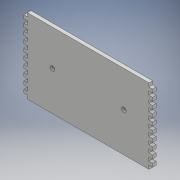
# Autodesk Inventor part: Base
Saved by Autodesk Inventor 2017 (Build 210142000, 142)
## iProperties
Created: 2017-04-26
Part Number: Base
Material: Generic
Document SubType Name: Modeling
Designer: Parshant Bombhi
Density: 1 g/cm^3
Appearance: Default
Author: Parshant Bombhi
Autodesk Inventor part; units mm, degrees
ref_plane "YZ Plane" through (0, 0, 0) normal (1, 0, 0) x (0, 1, 0)
ref_plane "XZ Plane" through (0, 0, 0) normal (0, 1, 0) x (-1, 0, 0)
ref_plane "XY Plane" through (0, 0, 0) normal (0, 0, 1) x (1, 0, 0)
sketch "Sketch5" plane through (0, 0, 0) normal (0, 1, 0) x (-1, 0, 0)
  circle A0 centre (177.8, -63.5) radius 3.9688
  circle A1 centre (50.8, -63.5) radius 3.9687
  line L0 (6.35, 0) -> (6.35, -6.35)
  line L1 (6.35, -6.35) -> (0, -6.35)
  line L2 (0, -6.35) -> (0, -12.7)
  line L3 (0, -12.7) -> (6.35, -12.7)
  line L4 (6.35, -12.7) -> (6.35, -19.05)
  line L5 (6.35, -19.05) -> (0, -19.05)
  line L6 (0, -19.05) -> (0, -25.4)
  line L7 (0, -25.4) -> (6.35, -25.4)
  line L8 (6.35, -25.4) -> (6.35, -31.75)
  line L9 (6.35, -31.75) -> (0, -31.75)
  line L10 (0, -31.75) -> (0, -38.1)
  line L11 (0, -38.1) -> (6.35, -38.1)
  line L12 (6.35, -38.1) -> (6.35, -44.45)
  line L13 (6.35, -44.45) -> (0, -44.45)
  line L14 (0, -44.45) -> (0, -50.8)
  line L15 (0, -50.8) -> (6.35, -50.8)
  line L16 (6.35, -50.8) -> (6.35, -57.15)
  line L17 (6.35, -57.15) -> (0, -57.15)
  line L18 (0, -57.15) -> (0, -63.5)
  line L19 (0, -63.5) -> (6.35, -63.5)
  line L20 (6.35, -63.5) -> (6.35, -69.85)
  line L21 (6.35, -69.85) -> (0, -69.85)
  line L22 (0, -69.85) -> (0, -76.2)
  line L23 (0, -76.2) -> (6.35, -76.2)
  line L24 (6.35, -76.2) -> (6.35, -82.55)
  line L25 (6.35, -82.55) -> (0, -82.55)
  line L26 (0, -82.55) -> (0, -88.9)
  line L27 (0, -88.9) -> (6.35, -88.9)
  line L28 (6.35, -88.9) -> (6.35, -95.25)
  line L29 (6.35, -95.25) -> (0, -95.25)
  line L30 (0, -95.25) -> (0, -101.6)
  line L31 (0, -101.6) -> (6.35, -101.6)
  line L32 (6.35, -101.6) -> (6.35, -107.95)
  line L33 (6.35, -107.95) -> (0, -107.95)
  line L34 (0, -107.95) -> (0, -114.3)
  line L35 (0, -114.3) -> (6.35, -114.3)
  line L36 (6.35, -114.3) -> (6.35, -120.65)
  line L37 (6.35, -120.65) -> (0, -120.65)
  line L38 (0, -120.65) -> (0, -127)
  line L39 (0, -127) -> (6.35, -127)
  line L40 (6.35, -127) -> (6.35, -133.35)
  line L41 (222.25, -133.35) -> (222.25, -127)
  line L42 (222.25, -127) -> (228.6, -127)
  line L43 (228.6, -127) -> (228.6, -120.65)
  line L44 (228.6, -120.65) -> (222.25, -120.65)
  line L45 (222.25, -120.65) -> (222.25, -114.3)
  line L46 (222.25, -114.3) -> (228.6, -114.3)
  line L47 (228.6, -114.3) -> (228.6, -107.95)
  line L48 (228.6, -107.95) -> (222.25, -107.95)
  line L49 (222.25, -107.95) -> (222.25, -101.6)
  line L50 (222.25, -101.6) -> (228.6, -101.6)
  line L51 (228.6, -101.6) -> (228.6, -95.25)
  line L52 (228.6, -95.25) -> (222.25, -95.25)
  line L53 (222.25, -95.25) -> (222.25, -88.9)
  line L54 (222.25, -88.9) -> (228.6, -88.9)
  line L55 (228.6, -88.9) -> (228.6, -82.55)
  line L56 (228.6, -82.55) -> (222.25, -82.55)
  line L57 (222.25, -82.55) -> (222.25, -76.2)
  line L58 (222.25, -76.2) -> (228.6, -76.2)
  line L59 (228.6, -76.2) -> (228.6, -69.85)
  line L60 (228.6, -69.85) -> (222.25, -69.85)
  line L61 (222.25, -69.85) -> (222.25, -63.5)
  line L62 (222.25, -63.5) -> (228.6, -63.5)
  line L63 (228.6, -63.5) -> (228.6, -57.15)
  line L64 (228.6, -57.15) -> (222.25, -57.15)
  line L65 (222.25, -57.15) -> (222.25, -50.8)
  line L66 (222.25, -50.8) -> (228.6, -50.8)
  line L67 (228.6, -50.8) -> (228.6, -44.45)
  line L68 (228.6, -44.45) -> (222.25, -44.45)
  line L69 (222.25, -44.45) -> (222.25, -38.1)
  line L70 (222.25, -38.1) -> (228.6, -38.1)
  line L71 (228.6, -38.1) -> (228.6, -31.75)
  line L72 (228.6, -31.75) -> (222.25, -31.75)
  line L73 (222.25, -31.75) -> (222.25, -25.4)
  line L74 (222.25, -25.4) -> (228.6, -25.4)
  line L75 (228.6, -25.4) -> (228.6, -19.05)
  line L76 (228.6, -19.05) -> (222.25, -19.05)
  line L77 (222.25, -19.05) -> (222.25, -12.7)
  line L78 (222.25, -12.7) -> (228.6, -12.7)
  line L79 (228.6, -12.7) -> (228.6, -6.35)
  line L80 (228.6, -6.35) -> (222.25, -6.35)
  line L81 (222.25, -6.35) -> (222.25, 0)
  line L82 (6.35, 0) -> (222.25, 0)
  line L83 (222.25, -133.35) -> (6.35, -133.35)
  point P0 (0, 0)
  dimension "Shaft_Diameter" = 7.9375
  dimension "d59" = 7.9375
  dimension "d73" = 6.35
  dimension "Teeth_Width" = 6.35
  dimension "d79" = 6.35
  dimension "d80" = 6.35
  dimension "d81" = 6.35
  dimension "d82" = 6.35
  dimension "d92" = 6.35
  dimension "d93" = 6.35
  dimension "d94" = 6.35
  dimension "d95" = 6.35
  dimension "d96" = 6.35
  dimension "d97" = 6.35
  dimension "d100" = 6.35
  dimension "d101" = 6.35
  dimension "d102" = 6.35
  dimension "d103" = 6.35
  dimension "d106" = 6.35
  dimension "d107" = 6.35
  dimension "d108" = 6.35
  dimension "d109" = 6.35
  dimension "d112" = 6.35
  dimension "d113" = 6.35
  dimension "d114" = 6.35
  dimension "d115" = 6.35
  dimension "d118" = 6.35
  dimension "d119" = 6.35
  dimension "d120" = 6.35
  dimension "d121" = 6.35
  dimension "d124" = 6.35
  dimension "d125" = 6.35
  dimension "d126" = 6.35
  dimension "d127" = 6.35
  dimension "d130" = 6.35
  dimension "d131" = 6.35
  dimension "d132" = 6.35
  dimension "d133" = 6.35
  dimension "d136" = 6.35
  dimension "d137" = 6.35
  dimension "d138" = 6.35
  dimension "d139" = 6.35
  dimension "d143" = 6.35
  dimension "d149" = 6.35
  dimension "d150" = 6.35
  dimension "d151" = 6.35
  dimension "d152" = 6.35
  dimension "d153" = 6.35
  dimension "d154" = 6.35
  dimension "d155" = 6.35
  dimension "d156" = 6.35
  dimension "d157" = 6.35
  dimension "d158" = 6.35
  dimension "d159" = 6.35
  dimension "d160" = 6.35
  dimension "d161" = 6.35
  dimension "d162" = 6.35
  dimension "d163" = 6.35
  dimension "d164" = 6.35
  dimension "d165" = 6.35
  dimension "d166" = 6.35
  dimension "d167" = 6.35
  dimension "d168" = 6.35
  dimension "d169" = 6.35
  constraints: 168 end point, 60 perpendicular, 11 horizontal, 11 vertical, 2 centre point
  measures "Shaft_Diameter" diameter of A0
  measures "d59" diameter of A1
  measures "d73" distance of L1.end L2.end
  measures "Teeth_Width" distance of L0.start L0.end
  measures "d79" distance between parallel lines of L0 L2
  measures "d80" distance of L5.end L6.end
  measures "d81" distance of L3.end L4.end
  measures "d82" distance between parallel lines of L4 L6
  measures "d92" distance of L6.end L7.end
  measures "d93" distance between parallel lines of L2 L4
  measures "d94" distance of L9.end L10.end
  measures "d95" distance of L7.end L8.end
  measures "d96" distance between parallel lines of L8 L10
  measures "d97" distance of L10.end L11.end
  measures "d100" distance of L13.end L14.end
  measures "d101" distance of L11.end L12.end
  measures "d102" distance between parallel lines of L12 L14
  measures "d103" distance of L14.end L15.end
  measures "d106" distance of L17.end L18.end
  measures "d107" distance of L15.end L16.end
  measures "d108" distance between parallel lines of L16 L18
  measures "d109" distance of L18.end L19.end
  measures "d112" distance of L21.end L22.end
  measures "d113" distance of L19.end L20.end
  measures "d114" distance between parallel lines of L20 L22
  measures "d115" distance of L22.end L23.end
  measures "d118" distance of L25.end L26.end
  measures "d119" distance of L23.end L24.end
  measures "d120" distance between parallel lines of L24 L26
  measures "d121" distance of L26.end L27.end
  measures "d124" distance of L29.end L30.end
  measures "d125" distance of L27.end L28.end
  measures "d126" distance between parallel lines of L28 L30
  measures "d127" distance of L30.end L31.end
  measures "d130" distance of L33.end L34.end
  measures "d131" distance of L31.end L32.end
  measures "d132" distance between parallel lines of L32 L34
  measures "d133" distance of L34.end L35.end
  measures "d136" distance of L37.end L38.end
  measures "d137" distance of L35.end L36.end
  measures "d138" distance between parallel lines of L36 L38
  measures "d139" distance of L38.end L39.end
  measures "d143" distance of L39.end L40.end
  measures "d149" distance of L43.start L44.start
  measures "d150" distance of L41.start L42.start
  measures "d151" distance between parallel lines of L41 L43
  measures "d152" distance of L47.start L47.end
  measures "d153" distance of L44.end L46.start
  measures "d154" distance between parallel lines of L45 L47
  measures "d155" distance of L47.end L48.end
  measures "d156" distance between parallel lines of L43 L45
  measures "d157" distance of L50.end L51.end
  measures "d158" distance of L48.end L49.end
  measures "d159" distance between parallel lines of L49 L51
  measures "d160" distance of L51.end L52.end
  measures "d161" distance of L54.end L56.start
  measures "d162" distance of L52.end L53.end
  measures "d163" distance between parallel lines of L53 L55
  measures "d164" distance of L56.start L56.end
  measures "d165" distance of L58.end L59.end
  measures "d166" distance of L56.end L58.start
  measures "d167" distance between parallel lines of L57 L59
  measures "d168" distance of L59.end L60.end
  measures "d169" distance of L63.start L63.end
extrude "Extrusion4" add sketch "Sketch5" along normal blind 6.35
equation "\"d59\" = Shaft_Diameter"
body "Solid2"
